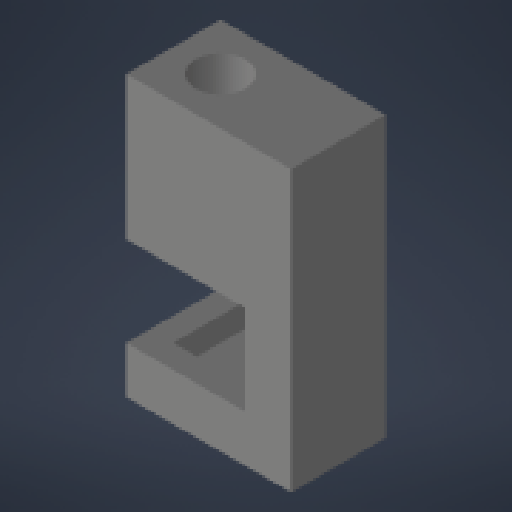
# Autodesk Inventor part: Adafruit_1528_4663-ND_House_01
Saved by Autodesk Inventor 2026.2 (Build 302298000, 298)
## iProperties
Created: 2026-02-03
Part Number: Adafruit_1528_4663-ND_House_01
Material: Generic
Document SubType Name: Modeling
Designer: vckot
Density: 1 g/cm^3
Appearance: Gray
Author: vckot
Autodesk Inventor part; units mm, degrees
ref_plane "YZ Plane" through (0, 0, 0) normal (1, 0, 0) x (0, 1, 0)
ref_plane "XZ Plane" through (0, 0, 0) normal (0, 1, 0) x (-1, 0, 0)
ref_plane "XY Plane" through (0, 0, 0) normal (0, 0, 1) x (1, 0, 0)
sketch "Sketch1" plane through (0, 0, 0) normal (0, 0, 1) x (1, 0, 0)
  line L0 (-6.25, -7.25) -> (6.25, -7.25)
  line L1 (6.25, -7.25) -> (6.25, 7.25)
  line L2 (6.25, 7.25) -> (-6.25, 7.25)
  line L3 (-6.25, 7.25) -> (-6.25, -7.25)
  line L4 (-6.25, -7.25) -> (6.25, 7.25) construction
  line L5 (6.25, -7.25) -> (-6.25, 7.25) construction
  line L6 (-8.75, -9.75) -> (8.75, -9.75)
  line L7 (8.75, -9.75) -> (8.75, 9.75)
  line L8 (8.75, 9.75) -> (-8.75, 9.75)
  line L9 (-8.75, 9.75) -> (-8.75, -9.75)
  line L10 (-8.75, -9.75) -> (8.75, 9.75) construction
  line L11 (8.75, -9.75) -> (-8.75, 9.75) construction
  line L12 (-3.75, -4.75) -> (3.75, -4.75)
  line L13 (3.75, -4.75) -> (3.75, 4.75)
  line L14 (3.75, 4.75) -> (-3.75, 4.75)
  line L15 (-3.75, 4.75) -> (-3.75, -4.75)
  line L16 (-3.75, -4.75) -> (3.75, 4.75) construction
  line L17 (3.75, -4.75) -> (-3.75, 4.75) construction
  point P0 (0, 0)
  dimension "d0" = 12.5
  dimension "d1" = 14.5
  dimension "d2" = 17.5
  dimension "d3" = 19.5
  dimension "d4" = 7.5
  dimension "d5" = 9.5
  constraints: 36 end point, 6 midpoint, 6 parallel, 3 horizontal, 3 perpendicular
  measures "d0" distance of L2.end L1.end
  measures "d1" distance of L1.end L0.end
  measures "d2" distance of L7.end L8.end
  measures "d3" distance of L6.end L7.end
  measures "d4" distance of L13.end L14.end
  measures "d5" distance of L12.end L13.end
extrude "Extrusion1" add sketch "Sketch1" along normal blind 2.5 contours L3 L2 L1 L0 | L9 L8 L7 L6
extrude "Extrusion2" add sketch "Sketch1" against normal blind 7.5 contours L9 L8 L7 L6
sketch "Sketch2" plane through (0, 0, 2.5) normal (0, 0, 1) x (1, 0, 0)
  line L0 (-8.75, -9.75) -> (-8.75, 9.75) projected
  line L1 (-3.75, -4.75) -> (-8.75, -4.75)
  line L2 (-8.75, -4.75) -> (-8.75, 4.75)
  line L3 (-8.75, 4.75) -> (-3.75, 4.75)
  line L4 (-3.75, 4.75) -> (-3.75, -4.75)
  line L5 (-3.75, -4.75) -> (-3.75, 4.75) projected
  point P0 (0, 0)
  point P1 (-3.75, 0)
  constraints: 8 end point, 2 midpoint, 2 parallel, 2 point on line, 1 horizontal, 1 perpendicular
extrude "Extrusion3" cut sketch "Sketch2" against normal through all
thicken "Thicken1" operation add thickness 10.199 both sides no extend neighbours no toward (0, 1, 0) faces at (2.9167, 9.75, -0.8333)
sketch "Sketch3" plane through (-8.75, 19.949, 2.5) normal (0, 1, 0) x (1, 0, 0)
  line L0 (0, 10) -> (0, 0) projected
  point P0 (8.75, 2.5)
  point P1 (5, 5)
  point P2 (0, 5)
  dimension "d22" = 5
  constraints: 1 horizontal alignment, 1 midpoint
  measures "d22" distance from line of L0 point (5, 5)
hole "Hole1" at (-3.75, 19.949, -2.5) direction (0, -1, 0) diameter 5.35 depth 10 tip angle 118
body "Solid1"
